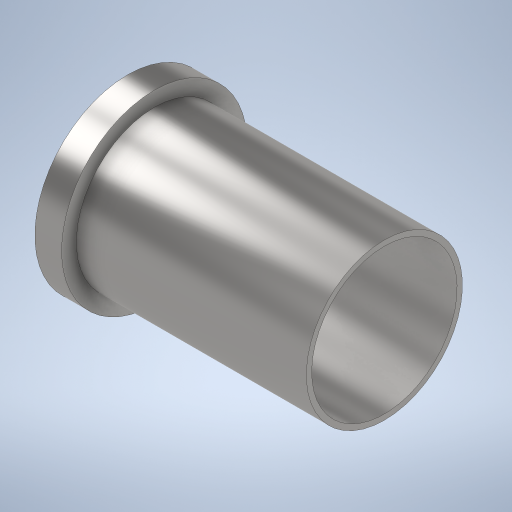
# Autodesk Inventor part: combustion chamber
Saved by Autodesk Inventor 2023 (Build 270158000, 158)
## iProperties
Created: 2022-09-14
Part Number: combustion chamber
Material: Stainless Steel, Austenitic
Document SubType Name: Modeling
Designer: station
Density: 8 g/cm^3
Appearance: Semi-Polished
Author: station
Autodesk Inventor part; units mm, degrees
ref_plane "YZ Plane" through (0, 0, 0) normal (1, 0, 0) x (0, 1, 0)
ref_plane "XZ Plane" through (0, 0, 0) normal (0, 1, 0) x (-1, 0, 0)
ref_plane "XY Plane" through (0, 0, 0) normal (0, 0, 1) x (1, 0, 0)
sketch "Sketch1" plane through (0, 0, 0) normal (0, 0, 1) x (1, 0, 0)
  line L0 (0, 0) -> (0, 54.375)
  line L1 (0, 54.375) -> (192, 54.375)
  line L2 (0, 0) -> (772.3927, 0)
  line L3 (253.9225, 18.624) -> (253.9225, 0) construction
  line L4 (192, 54.375) -> (253.9225, 18.624)
  line L5 (253.9225, 18.624) -> (256.9225, 18.624)
  line L6 (256.9225, 18.624) -> (325.3908, 36.97)
  line L7 (325.3908, 36.97) -> (325.3908, 0)
  line L8 (192, 54.375) -> (192, 0)
  line L9 (0, 54.375) -> (0, 69.375)
  line L10 (0, 69.375) -> (20, 69.375)
  line L11 (20, 69.375) -> (20, 58.375)
  line L12 (192, 54.375) -> (192, 74.375)
  line L13 (20, 58.375) -> (172, 58.375)
  line L14 (172, 58.375) -> (192, 58.375)
  dimension "d9" = 54.375
  dimension "d10" = 192
  dimension "d12" = 18.624
  dimension "d13" = 150
  dimension "d15" = 3
  dimension "d16" = 15
  dimension "d17" = 36.97
  dimension "d18" = 518.4701
  dimension "d19" = 15
  dimension "d20" = 20
  dimension "d21" = 11
  constraints: 30 end point, 7 perpendicular, 4 point on line, 2 horizontal, 2 vertical, 1 parallel
  measures "d9" distance of L0.start L0.end
  measures "d10" distance of L0.end L1.end
  measures "d12" distance of L3.start L3.end
  measures "d13" angle of L4 L1
  measures "d15" distance of L3.start L5.end
  measures "d16" angle of L2 L6
  measures "d17" distance of L6.end L7.end
  measures "d18" distance from line of L2.end L3
  measures "d19" distance of L0.end L9.end
  measures "d20" distance of L9.end L10.end
  measures "d21" distance of L10.end L11.end
revolve "Revolution2" add sketch "Sketch1" angle 360 about axis through (0, 0, 0) along (1, 0, 0) contours L9 L10 L11 L13 L14 L12 L1
body "Solid2"
